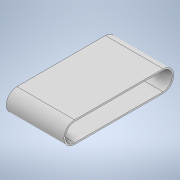
# Autodesk Inventor part: Shooting_Belt
Saved by Autodesk Inventor 2020 (Build 240168000, 168)
## iProperties
Created: 2022-01-26
Part Number: Shooting_Belt
Material: Generic
Document SubType Name: Modeling
Designer: danie
Density: 1 g/cm^3
Appearance: Default
Author: danie
Autodesk Inventor part; units mm, degrees
ref_plane "YZ Plane" through (0, 0, 0) normal (1, 0, 0) x (0, 1, 0)
ref_plane "XZ Plane" through (0, 0, 0) normal (0, 1, 0) x (-1, 0, 0)
ref_plane "XY Plane" through (0, 0, 0) normal (0, 0, 1) x (1, 0, 0)
sketch "Sketch1" plane through (0, 0, 0) normal (1, 0, 0) x (0, 1, 0)
  line L0 (0, 0) -> (0, 194.818) construction
  line L1 (20.32, 0) -> (20.32, 194.818)
  line L2 (-20.32, 194.818) -> (-20.32, 0)
  arc A0 (-20.32, 0) -> (20.32, 0) centre (0, 0) ccw
  arc A1 (20.32, 194.818) -> (-20.32, 194.818) centre (0, 194.818) ccw
  line L3 (23.495, 194.818) -> (23.495, 0)
  arc A2 (-23.495, 0) -> (23.495, 0) centre (0, 0) ccw
  line L4 (-23.495, 0) -> (-23.495, 194.818)
  arc A3 (23.495, 194.818) -> (-23.495, 194.818) centre (0, 194.818) ccw
  point P0 (0, 97.409)
  dimension "d0" = 194.818
  dimension "d1" = 40.64
  dimension "d2" = 3.175
  constraints: 12 end point, 8 point on circle, 4 centre point, 4 tangent, 2 parallel, 1 midpoint, 1 vertical, 3 other
  measures "d0" distance of L0.start L0.end
  measures "d1" diameter of A1
  measures "d2" distance between parallel lines of L1 L3
extrude "Extrusion1" add sketch "Sketch1" along normal blind 127
body "Solid1"
